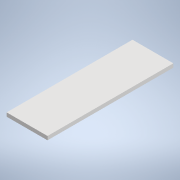
# Autodesk Inventor part: Back
Saved by Autodesk Inventor 2021 (Build 250183000, 183)
## iProperties
Created: 2020-07-16
Part Number: Back
Material: Generic
Document SubType Name: Modeling
Designer: adick
Density: 1 g/cm^3
Appearance: Default
Author: adick
Autodesk Inventor part; units mm, degrees
ref_plane "YZ Plane" through (0, 0, 0) normal (1, 0, 0) x (0, 1, 0)
ref_plane "XZ Plane" through (0, 0, 0) normal (0, 1, 0) x (-1, 0, 0)
ref_plane "XY Plane" through (0, 0, 0) normal (0, 0, 1) x (1, 0, 0)
sketch "Sketch1" plane through (0, 0, 0) normal (0, 0, 1) x (1, 0, 0)
  line L0 (-69.85, 132.5) -> (-69.85, -132.5) projected
  line L1 (69.85, 132.5) -> (-69.85, 132.5)
  line L2 (-69.85, 132.5) -> (-69.85, 119.8)
  line L3 (-69.85, 119.8) -> (69.85, 119.8)
  line L4 (69.85, 119.8) -> (69.85, 132.5)
  point P0 (0, 0)
  point P1 (69.85, 111.3788)
  point P2 (-57.15, -132.5)
  point P3 (-57.15, -68.2625)
  constraints: 8 end point, 2 parallel, 1 horizontal, 1 perpendicular, 6 other
extrude "Extrusion1" add sketch "Sketch1" along normal blind 430
body "Solid1"
